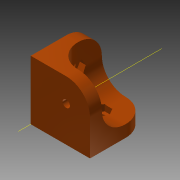
# Autodesk Inventor part: corner tab
Saved by Autodesk Inventor 2013 (Build 170138000, 138)
## iProperties
Created: 2013-07-28
Part Number: corner tab
Material: Generic
Document SubType Name: Modeling
Designer: employee
Density: 1 g/cm^3
Mass: 8.15402 g
Surface Area: 35.3481 cm^2
Volume: 8.15402 cm^3
Author: employee
Autodesk Inventor part; units mm, degrees
ref_plane "YZ Plane" through (0, 0, 0) normal (1, 0, 0) x (0, 1, 0)
ref_plane "XZ Plane" through (0, 0, 0) normal (0, 1, 0) x (-1, 0, 0)
ref_plane "XY Plane" through (0, 0, 0) normal (0, 0, 1) x (1, 0, 0)
sketch "Sketch1" plane through (0, 0, 0) normal (0, 0, 1) x (1, 0, 0)
  line L0 (0, 0) -> (25, 0)
  line L1 (25, 0) -> (25, 25)
  line L2 (25, 25) -> (0, 25)
  line L3 (0, 25) -> (0, 0)
  dimension "d0" = 25
  constraints: 8 end point, 2 parallel, 2 perpendicular, 1 coincident, 1 horizontal
  measures "d0" distance of L0.start L0.end
extrude "Extrusion1" add sketch "Sketch1" along normal blind 5
sketch "Sketch2" plane through (0, 0, 0) normal (0, -1, 0) x (1, 0, 0)
  line L0 (0, 0) -> (25, 0) projected
  line L1 (25, 0) -> (25, 5) projected
  line L2 (0, 5) -> (25, 5) projected
  line L3 (0, 0) -> (0, 5) projected
  line L4 (0, 0) -> (25, 0)
  line L5 (25, 0) -> (25, 25)
  line L6 (25, 25) -> (0, 25)
  line L7 (0, 25) -> (0, 0)
  constraints: 8 end point, 2 parallel, 2 perpendicular, 1 horizontal
extrude "Extrusion2" add sketch "Sketch2" against normal blind 5 contours L7 L6 L5 L2
sketch "Sketch3" plane through (0, 0, 0) normal (-1, 0, 0) x (0, 0, 1)
  line L0 (5, 25) -> (25, 25)
  line L1 (25, 25) -> (25, 5)
  line L2 (25, 5) -> (5, 5)
  line L3 (5, 5) -> (5, 25)
  constraints: 8 end point, 2 parallel, 1 horizontal, 1 perpendicular
extrude "Extrusion3" add sketch "Sketch3" against normal blind 5
fillet "Fillet2" radius 10 6 edges at (5, 5, 15) (5, 15, 5) (15, 5, 5) (2.5, 25, 25) (25, 2.5, 25) (25, 25, 2.5)
sketch "Sketch6" plane through (0, 5, 0) normal (0, 1, 0) x (1, 0, 0)
  arc A0 (15, -25) -> (25, -15) centre (15, -15) ccw projected
  circle A1 centre (15, -15) radius 1.55
  point P0 (0, 0)
  dimension "d20" = 3.1
  constraints: 1 centre point, 1 coincident
  measures "d20" diameter of A1
extrude "Extrusion6" cut sketch "Sketch6" along normal through all both and the other way through all
sketch "Sketch7" plane through (0, 5, 0) normal (0, 1, 0) x (1, 0, 0)
  line L0 (15, -25) -> (15, -16.55) projected
  arc A0 (15, -25) -> (25, -15) centre (15, -15) ccw projected
  line L1 (15, -18.2332) -> (12.2, -16.6166)
  line L2 (12.2, -16.6166) -> (12.2, -13.3834)
  line L3 (12.2, -13.3834) -> (15, -11.7668)
  line L4 (15, -11.7668) -> (17.8, -13.3834)
  line L5 (17.8, -13.3834) -> (17.8, -16.6166)
  line L6 (17.8, -16.6166) -> (15, -18.2332)
  point P0 (0, 0)
  dimension "d24" = 5.6
  constraints: 12 end point, 1 coincident, 1 point on line, 13 other
  measures "d24" distance between parallel lines of L5 L2
extrude "Extrusion7" cut sketch "Sketch7" along normal mid plane 5
pattern_circular "Circular Pattern2" count 3 over 360 about axis through (0, 0, 0) along (0.5774, 0.5774, 0.5774) of "Extrusion7", "Extrusion6"
body "Solid1"
